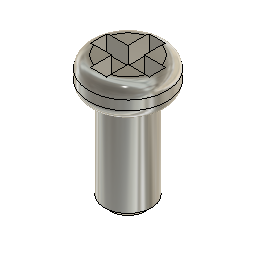
ottodiy-v129 (Autodesk Fusion 360 archive; units mm, degrees)
design "Screw_short"
Autodesk Fusion 360 part; units mm, degrees
note: some values were not read from the file. Chosen so that the rebuilt part matches the saved one: which face or edge a step refers to; a direction; the sign of a taper. Set by a fixed rule: which sketch regions a step uses.
cylinder "CylinderPrimitive1" add diameter 2 height 4 placed x (1, 0, 0) y (0, 1, 0) z (0, 0, 1) at (0, 0, 0)
cylinder "CylinderPrimitive2" add diameter 3.3 height 1.4 placed x (1, 0, 0) y (0, 1, 0) z (0, 0, 1) at (0, 0, 4)
fillet "Fillet1" radius 0.5 2 edges at (-1.5383, -0.5967, 5.4) (-1.5383, 0.5967, 4)
sketch "Sketch3" plane through (0, 0, 5.4) normal (0, 0, 1) x (-1, 0, 0)
  line L0 (-1.2532, 0.3491) -> (-1.2532, -0.3509)
  line L1 (1.2468, -0.3473) -> (1.2468, 0.3491)
  line L2 (1.2468, 0.3491) -> (-1.2532, -0.3509) construction
  line L3 (-1.2532, 0.3491) -> (1.2468, -0.3473) construction
  line L4 (-0.35, -1.25) -> (0.35, -1.25)
  line L5 (0.35, 1.25) -> (-0.35, 1.25)
  line L6 (-0.35, -1.25) -> (0.35, 1.25) construction
  line L7 (0.35, -1.25) -> (-0.35, 1.25) construction
  line L8 (0.35, -1.25) -> (0.35, -0.3509)
  line L9 (0.35, 0.3491) -> (0.35, 1.25)
  line L10 (1.2468, 0.3491) -> (0.35, 0.3491)
  line L11 (-0.35, 0.3491) -> (-1.2532, 0.3491)
  line L12 (-0.35, 1.25) -> (-0.35, 0.3491)
  line L13 (-0.35, -0.3509) -> (-0.35, -1.25)
  line L14 (-1.2532, -0.3509) -> (-0.35, -0.3509)
  line L15 (0.35, -0.3509) -> (1.2468, -0.3473)
  circle A0 centre (0, 0) radius 1.15
  dimension "d6" = 2.5
  dimension "d7" = 0.7
  dimension "d8" = 0.7
  dimension "d9" = 2.5
  constraint perpendicular L0 L10
  constraint parallel L10 L14
  constraint parallel L0 L1
  constraint horizontal L10
  constraint coincident L2 A0.centre
  constraint coincident L3 A0.centre
  constraint coincident A0.centre origin
  constraint perpendicular L4 L8
  constraint parallel L4 L5
  constraint parallel L8 L12
  constraint horizontal L4
  constraint coincident L6 A0.centre
  constraint coincident L7 A0.centre
  constraint coincident L8.end L14
  constraint collinear L10 L11
  constraint vertical L4.start L5.end
  measures "d6" distance of L0.end L1.start
  measures "d7" distance of L0.start L0.end
  measures "d8" distance of L5.start L5.end
  measures "d9" distance of L4.end L5.start
extrude "Extrude1" cut sketch "Sketch3" against normal blind 0.75 contours L0 L11 L14 A0 | L8 L9 L10 L11 L12 L13 L14 L15 A0 | L5 L9 L12 A0 | L4 L8 L13 A0 | L1 L10 L15 A0
chamfer "Chamfer1" distance 0.25 angle 45 1 edges at (-0.9323, 0.3616, 0)

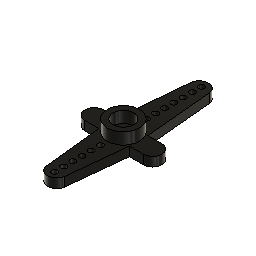
design "Servo_SG90_cross"
Autodesk Fusion 360 part; units mm, degrees
sketch "Sketch1" plane through (0, 0, 0) normal (0, 0, 1) x (1, 0, 0)
  circle A0 centre (0, 0) radius 3.5
  circle A1 centre (0, 0) radius 2.25
  circle A2 centre (0, 16.5) radius 2
  circle A3 centre (0, -14.5) radius 2
  circle A4 centre (-6.375, 0) radius 2
  circle A5 centre (6.375, 0) radius 2
  line L0 (0, 0) -> (0, 16.5) construction
  line L1 (-1.9917, 16.6818) -> (-3.4855, 0.3182)
  line L2 (-1.9893, -14.7069) -> (-3.4812, -0.3621)
  line L3 (1.9917, 16.6818) -> (3.4855, 0.3182)
  line L4 (1.9893, -14.7069) -> (3.4812, -0.3621)
  line L5 (-6.375, 2) -> (6.375, 2)
  line L6 (6.375, 2) -> (6.375, -2) construction
  line L7 (6.375, -2) -> (-6.375, -2)
  line L8 (-6.375, -2) -> (-6.375, 2) construction
  circle A6 centre (0, 0) radius 1.25
  circle A7 centre (0, 5) radius 0.625
  circle A8 centre (0, -5) radius 0.625
  point P0 (0, -16.5)
  point P1 (0, 18.5)
  point P2 (-8.375, 0)
  point P3 (8.375, 0)
  dimension "d1" = 7
  dimension "d2" = 4.5
  dimension "d5" = 35
  dimension "d7" = 4
  dimension "d8" = 16.75
  dimension "d9" = 14.5
  dimension "d12" = 2.5
  dimension "d14" = 5
  dimension "d15" = 1.25
  dimension "d22" = 5
  constraint coincident A0.centre A1.centre
  constraint vertical A0.centre A3.centre
  constraint vertical A0.centre A2.centre
  constraint coincident A3 P0
  constraint coincident A2 P1
  constraint vertical A3.centre P0
  constraint equal A2 A3
  constraint equal A3 A4
  constraint equal A3 A5
  constraint horizontal A0.centre A5.centre
  constraint coincident A4 P2
  constraint coincident A5 P3
  constraint horizontal A4.centre P2
  constraint horizontal A5.centre P3
  constraint coincident A2.centre L0.end
  constraint symmetric P2 P3 L0
  constraint coincident A2 L1.start
  constraint coincident A0 L1.end
  constraint tangent A2 L1
  constraint tangent A0 L1
  constraint coincident A3 L2.start
  constraint coincident A0 L2.end
  constraint tangent A3 L2
  constraint tangent A0 L2
  constraint symmetric L0 L1.start L3.start
  constraint symmetric L0 L1.end L3.end
  constraint symmetric L0 L2.start L4.start
  constraint symmetric L0 L2.end L4.end
  constraint horizontal L5
  constraint vertical L6
  constraint horizontal L7
  constraint vertical L8
  constraint coincident A5 L6.end
  constraint coincident A4 L5.start
  constraint coincident A5.centre L6
  constraint coincident A4.centre L8
  constraint coincident L0 A7.centre
  constraint equal A7 A8
  constraint vertical A0.centre A8.centre
  measures "d1" diameter of A0
  measures "d2" diameter of A1
  measures "d5" distance of P0 P1
  measures "d7" diameter of A3
  measures "d8" horizontal distance of P2 P3
  measures "d9" distance of A0.centre A3.centre
  measures "d12" diameter of A6
  measures "d14" distance of A0.centre A7.centre
  measures "d15" diameter of A7
  measures "d22" distance of A0.centre A8.centre
extrude "Extrude1" add sketch "Sketch1" along normal blind 2.5 contours A0 A1 L5 L7 | A0 A1 L5 | A0 A1 L7 | A0 A1 L5 L7
extrude "Extrude2" add sketch "Sketch1" against normal blind 2 contours A0 A1 L5 L7 | A0 A5 L3 L4 L5 L7 | A0 L3 L5 | A0 L4 L7 | A0 A1 L5 | A0 A2 L1 L3 L5 | A0 A3 L2 L4 L7 | A0 A1 L7 | A0 A1 L5 L7 | A0 L1 L5 | A1 L5 | A1 L5 L7 | A2 | A5 | A0 L2 L7 | A1 L7 | A3 | A0 A4 L1 L2 L5 L7 | A4 | A6 | A7 | A8
extrude "Extrude4" cut sketch "Sketch1" against normal through all contours A7
pattern_linear "R-Pattern1" count 7 spacing 2 along (0, 1, 0) of "Extrude4"
extrude "Extrude5" cut sketch "Sketch1" against normal through all contours A8
pattern_linear "R-Pattern2" count 6 spacing 2 along (0, -1, 0) of "Extrude5"
extrude "Extrude6" cut sketch "Sketch1" against normal through all contours A6

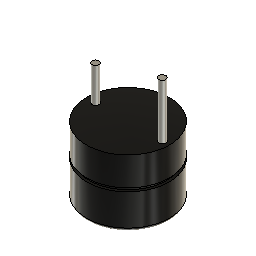
design "Buzzer"
Autodesk Fusion 360 part; units mm, degrees
cylinder "CylinderPrimitive1" add diameter 12 height 9.7 placed x (1, 0, 0) y (0, 1, 0) z (0, 0, 1) at (0, 0, 0)
fillet "Fillet1" radius 0.5 1 edges at (-5.594, 2.1697, 0)
cylinder "CylinderPrimitive2" add diameter 1 height 5 placed x (1, 0, 0) y (0, 1, 0) z (0, 0, 1) at (-4.7065, 0, 9.7)
cylinder "CylinderPrimitive3" add diameter 1 height 8 placed x (1, 0, 0) y (0, 1, 0) z (0, 0, 1) at (5, 0, 9.7)
hole "Hole1" at (0, 0, 0) direction (0, 0, 1) diameter 2 depth 5 tip angle 118
sketch "Sketch6" plane through (0, 0, 0) normal (0, 0, -1) x (1, 0, 0)
  circle A0 centre (0, 0) radius 1
  circle A1 centre (0, 0) radius 5.5
  circle A2 centre (4.1669, 0) radius 1.0832
  circle A3 centre (4.1669, 0) radius 0.7697
  line L0 (4.3232, 0.5982) -> (4.0106, 0.5982)
  line L1 (4.0106, 0.5982) -> (4.0106, -0.5982)
  line L2 (4.0106, -0.5982) -> (4.3232, -0.5982)
  line L3 (4.3232, -0.5982) -> (4.3232, 0.5982)
  line L4 (4.3232, 0.5982) -> (4.0106, -0.5982) construction
  line L5 (4.0106, 0.5982) -> (4.3232, -0.5982) construction
  line L6 (4.7651, -0.1703) -> (3.5686, -0.1703)
  line L7 (3.5686, -0.1703) -> (3.5686, 0.1703)
  line L8 (3.5686, 0.1703) -> (4.7651, 0.1703)
  line L9 (4.7651, 0.1703) -> (4.7651, -0.1703)
  line L10 (4.7651, -0.1703) -> (3.5686, 0.1703) construction
  line L11 (3.5686, -0.1703) -> (4.7651, 0.1703) construction
  point P0 (4.1669, 0)
  point P1 (4.1669, 0)
  constraint concentric A2 A3
  constraint perpendicular L0 L1
  constraint parallel L0 L2
  constraint parallel L1 L3
  constraint horizontal L0
  constraint coincident L4 P1
  constraint coincident L5 P1
  constraint coincident P1 P0
  constraint perpendicular L6 L7
  constraint parallel L6 L8
  constraint parallel L7 L9
  constraint horizontal L6
  constraint coincident L10 P1
  constraint coincident L11 P1
  constraint equal L3 L8
extrude "Extrude1" cut sketch "Sketch6" against normal blind 0.25 contours A2 | L0 L1 L3 L8 | L3 L6 L8 L9 | L1 L3 L6 L8 | L1 L6 L7 L8 | L1 L2 L3 L6
sketch "Sketch9" plane through (0, 0, 0) normal (0, 1, 0) x (1, 0, 0)
  line L0 (6.1265, -5.5653) -> (5.6265, -5.5653)
  line L1 (5.6265, -5.5653) -> (5.6265, -5.0653)
  line L2 (5.6265, -5.0653) -> (6.1265, -5.0653)
  line L3 (6.1265, -5.0653) -> (6.1265, -5.5653)
  dimension "d13" = 0.5
  dimension "d14" = 0.5
  constraint horizontal L0
  constraint vertical L1
  constraint horizontal L2
  constraint vertical L3
  measures "d13" distance of L0.start L0.end
  measures "d14" distance of L0.start L2.end
revolve "Revolve1" cut sketch "Sketch9" angle 360 about axis through (0, 0, 1.75) along (0, 0, 1)

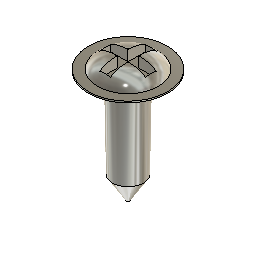
design "Screw_pointed"
Autodesk Fusion 360 part; units mm, degrees
cylinder "CylinderPrimitive1" add diameter 2 height 7.5 placed x (1, 0, 0) y (0, 1, 0) z (0, 0, 1) at (0, 0, 0)
cylinder "CylinderPrimitive2" add diameter 4 height 0.75 placed x (1, 0, 0) y (0, 1, 0) z (0, 0, 1) at (0, 0, 7.5)
fillet "Fillet1" radius 1.75 1 edges at (-1.8647, -0.7232, 8.25)
sketch "Sketch3" plane through (0, 0, 8.25) normal (0, 0, 1) x (-1, 0, 0)
  circle A0 centre (0, 0) radius 0.5639
  line L0 (-1.5, 0.35) -> (-1.5, -0.35)
  line L1 (1.5, -0.35) -> (1.5, 0.35)
  line L2 (1.5, 0.35) -> (-1.5, -0.35) construction
  line L3 (-1.5, 0.35) -> (1.5, -0.35) construction
  line L4 (-0.35, -1.5) -> (0.35, -1.5)
  line L5 (0.35, 1.5) -> (-0.35, 1.5)
  line L6 (-0.35, -1.5) -> (0.35, 1.5) construction
  line L7 (0.35, -1.5) -> (-0.35, 1.5) construction
  line L8 (0.35, -1.5) -> (0.35, -0.35)
  line L9 (0.35, 0.35) -> (0.35, 1.5)
  line L10 (1.5, 0.35) -> (0.35, 0.35)
  line L11 (-0.35, 0.35) -> (-1.5, 0.35)
  line L12 (-0.35, 1.5) -> (-0.35, 0.35)
  line L13 (-0.35, -0.35) -> (-0.35, -1.5)
  line L14 (-1.5, -0.35) -> (-0.35, -0.35)
  line L15 (0.35, -0.35) -> (1.5, -0.35)
  dimension "d6" = 3
  dimension "d7" = 0.7
  dimension "d8" = 0.7
  dimension "d9" = 3
  constraint perpendicular L0 L10
  constraint parallel L10 L14
  constraint parallel L0 L1
  constraint horizontal L10
  constraint coincident L2 A0.centre
  constraint coincident L3 A0.centre
  constraint coincident A0.centre origin
  constraint perpendicular L4 L8
  constraint parallel L4 L5
  constraint parallel L8 L12
  constraint horizontal L4
  constraint coincident L6 A0.centre
  constraint coincident L7 A0.centre
  constraint coincident L8.end L14
  constraint collinear L10 L11
  measures "d6" distance of L0.end L1.start
  measures "d7" distance of L0.start L0.end
  measures "d8" distance of L5.start L5.end
  measures "d9" distance of L4.end L5.start
extrude "Extrude1" cut sketch "Sketch3" against normal blind 0.7 contours A0 L8 L9 L10 L11 L12 L13 L14 L15 | A0 L1 L10 L15 | A0 L5 L9 L12 | A0 L4 L8 L13 | A0 L0 L11 L14
draft "Draft1" angle -1 neutral plane through (0, 0, 0) pull (0, 0, 1) 1 faces at (0.995, -0.0996, 2.5)
chamfer "Chamfer1" distance 0.9 distance2 1.5 1 edges at (-0.9323, 0.3616, 0) measured on face at (-0.3296, 0.5031, 0)
cylinder "CylinderPrimitive3" add diameter 5.2 height 0.1 placed x (0, 1, 0) y (1, 0, 0) z (0, 0, -1) at (0, 0, 7.5)
